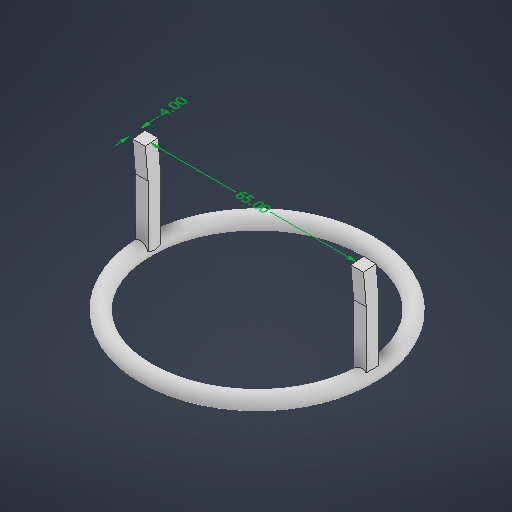
# Autodesk Inventor part: Basket Holder 2
Saved by Autodesk Inventor 2026.2 (Build 302298010, 298A)
## iProperties
Created: 2026-04-15
Part Number: Basket Holder 2
Material: Generic
Document SubType Name: Modeling
Designer: lenovo
Density: 1 g/cm^3
Appearance: Default
Author: lenovo
## iProperties of the stored document Basket Holder 2 _3DPrint.ipt
Created: 2026-04-17
Part Number: Basket Holder 2 _3DPrint
Material: Generic
Document SubType Name: Modeling
Designer: lenovo
Density: 1 g/cm^3
Appearance: Default
Author: lenovo
Autodesk Inventor part; units mm, degrees
ref_plane "YZ Plane" through (0, 0, 0) normal (1, 0, 0) x (0, 1, 0)
ref_plane "XZ Plane" through (0, 0, 0) normal (0, 1, 0) x (-1, 0, 0)
ref_plane "XY Plane" through (0, 0, 0) normal (0, 0, 1) x (1, 0, 0)
sketch "Sketch1" plane through (0, 0, 0) normal (0, 0, 1) x (1, 0, 0)
  circle A0 centre (-35, 0) radius 2.5
  line L0 (0, -2.5) -> (0, 2.5) construction
  point P0 (0, 0)
  dimension "d0" = 5
  dimension "d1" = 5
  dimension "d26" = 35
  constraints: 2 end point, 1 centre point, 1 midpoint, 1 vertical
  measures "d0" diameter of A0
  measures "d1" distance of L0.start L0.end
  measures "d26" distance from line of L0 A0.centre
revolve "Revolution1" add sketch "Sketch1" angle 360 about axis through (0, -2.5, 0) along (0, 1, 0)
sketch "Sketch2" plane through (0, 0, 0) normal (0, 1, 0) x (-1, 0, 0)
  circle A0 centre (0, 0) radius 32.5 projected
  line L0 (36.5, 2) -> (32.5, 2)
  line L1 (32.5, 2) -> (32.5, -2)
  line L2 (32.5, -2) -> (36.5, -2)
  line L3 (36.5, -2) -> (36.5, 2)
  line L4 (36.5, 2) -> (32.5, -2) construction
  line L5 (32.5, 2) -> (36.5, -2) construction
  line L6 (-32.5, 2) -> (-36.5, 2)
  line L7 (-36.5, 2) -> (-36.5, -2)
  line L8 (-36.5, -2) -> (-32.5, -2)
  line L9 (-32.5, -2) -> (-32.5, 2)
  line L10 (-32.5, 2) -> (-36.5, -2) construction
  line L11 (-36.5, 2) -> (-32.5, -2) construction
  point P0 (34.5, 0)
  point P1 (-34.5, 0)
  point P2 (32.5, 0)
  dimension "d5" = 4
  dimension "d6" = 4
  dimension "d7" = 4
  dimension "d8" = 4
  dimension "d31" = 32.5
  dimension "d32" = 32.5
  constraints: 24 end point, 5 midpoint, 4 parallel, 2 horizontal, 2 perpendicular
  measures "d5" distance of L2.end L1.end
  measures "d6" distance of L1.end L0.end
  measures "d7" distance of L8.end L7.end
  measures "d8" distance of L7.end L6.end
  measures "d31" distance from line of point (0, 0) L9
  measures "d32" distance of point (0, 0) point (32.5, 0)
extrude "Extrusion1" add sketch "Sketch2" along normal blind 20 contours L9 L8 L7 L6 | L1 L0 L3 L2
sketch "Sketch3" plane through (36.5, 1.9577, -2) normal (1, 0, 0) x (0, 0, -1)
  line L0 (0, 18.0423) -> (-4, 18.0423) projected
  line L1 (-4, 18.0423) -> (-4.8716, 28.0042)
  line L2 (-4, 18.0423) -> (6, 18.0423) construction
  line L3 (-4.8716, 28.0042) -> (-0.8868, 28.3528)
  line L4 (-0.8868, 28.3528) -> (0, 18.0423)
  point P0 (-2, -1.9577)
  dimension "d9" = 10
  dimension "d10" = 95
  dimension "d11" = 4
  constraints: 8 end point, 1 equal length, 1 horizontal, 1 perpendicular
  measures "d9" distance of L0.end L1.end
  measures "d10" angle of L2 L1
  measures "d11" distance of L1.end L3.end
extrude "Extrusion2" add sketch "Sketch3" against normal blind 73
extrude "Extrusion3" cut sketch "Sketch3" against normal blind 59
extrude "Extrusion4" add sketch "Sketch3" against normal blind 4
extrude "Extrusion6" cut sketch "Sketch3" against normal blind 69
extrude "Extrusion7" add sketch "Sketch3" against normal blind 4
body "Solid1"
